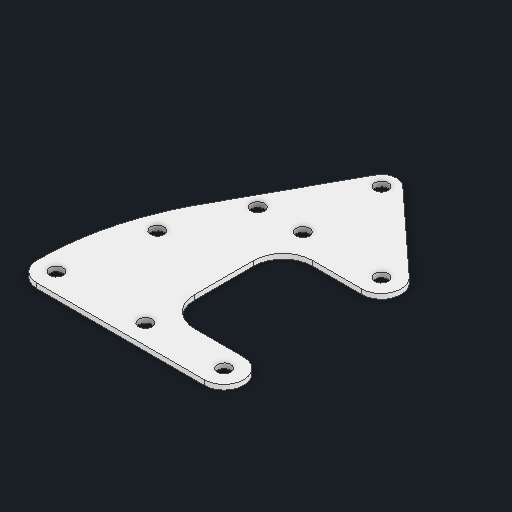
# Autodesk Inventor part: Funnel Gusset Back Improved V2
Saved by Autodesk Inventor 2025.1 (Build 291241000, 241)
## iProperties
Created: 2024-10-23
Part Number: Funnel Gusset Back Improved V2
Material: Acetal Resin, White
Document SubType Name: Modeling
Designer: avere
Density: 1.425 g/cm^3
Appearance: Smooth - White
Author: avere
Autodesk Inventor part; units mm, degrees
ref_plane "YZ Plane" through (0, 0, 0) normal (1, 0, 0) x (0, 1, 0)
ref_plane "XZ Plane" through (0, 0, 0) normal (0, 1, 0) x (-1, 0, 0)
ref_plane "XY Plane" through (0, 0, 0) normal (0, 0, 1) x (1, 0, 0)
sketch "main" plane through (0, 0, 0) normal (0, 0, 1) x (1, 0, 0)
  line L0 (12.0188, -14.2552) -> (33.1027, 24.2387)
  circle A0 centre (21.9619, 13.8124) radius 2.1844
  circle A1 centre (31.5972, 36.5815) radius 2.1844
  circle A2 centre (36.4896, 64.2776) radius 2.1844
  line L1 (36.4904, 70.6276) -> (-17.6528, 70.6344)
  circle A3 centre (7.7473, 64.2844) radius 2.1844
  line L2 (7.7507, 48.4162) -> (7.7558, 29.3619)
  arc A4 (7.7507, 48.4162) -> (-1.7768, 57.9386) centre (-1.7743, 48.4136) ccw
  arc A5 (-1.7692, 19.8344) -> (7.7558, 29.3619) centre (-1.7692, 29.3594) ccw
  line L3 (-17.645, 57.9344) -> (-1.7768, 57.9386)
  arc A6 (-17.6528, 70.6344) -> (-17.645, 57.9344) centre (-17.645, 64.2844) ccw
  arc A7 (-17.6527, 19.8344) -> (-21.9541, 8.8131) centre (-17.6527, 13.4844) ccw
  circle A8 centre (7.7473, 13.4844) radius 2.1844
  line L4 (-1.7692, 19.8344) -> (-17.6527, 19.8344)
  arc A9 (4.4483, -15.4983) -> (12.0188, -14.2552) centre (7.7473, -11.9156) ccw
  line L5 (4.4483, -15.4983) -> (-21.9541, 8.8131)
  circle A10 centre (7.7473, -11.9156) radius 2.1844
  circle A11 centre (-17.645, 64.2844) radius 2.1844
  circle A12 centre (-17.6527, 13.4844) radius 2.1844
  arc A13 (42.8396, 64.2776) -> (36.4904, 70.6276) centre (36.4896, 64.2776) ccw
  arc A14 (33.1027, 24.2387) -> (42.8396, 64.2776) centre (-44.3506, 64.2776) ccw
  point P0 (10.5119, 26.5593)
  dimension "d1" = 9.7405
  dimension "d2" = 4.3688
  dimension "d3" = 4.3688
  dimension "d4" = 4.3688
  dimension "d5" = 4.3688
  dimension "d6" = 4.3688
  dimension "d10" = 50.8
  dimension "d11" = 50.8
  dimension "d13" = 6.35
  measures "d1" diameter of A9
  measures "d2" diameter of A2
  measures "d3" diameter of A3
  measures "d4" diameter of A1
  measures "d5" diameter of A0
  measures "d6" diameter of A8
  measures "d10" distance of A7.centre A11.centre
  measures "d11" distance of A8.centre A3.centre
  measures "d13" radius of A6
sketch "Sketch1" plane through (0, 0, 0) normal (0, 1, 0) x (-1, 0, 0)
  line L0 (29.6638, -78.5396) -> (50.7478, -40.0457)
  circle A0 centre (39.607, -50.472) radius 2.1844
  circle A1 centre (49.2422, -27.7029) radius 2.1844
  circle A2 centre (54.1346, -0.0068) radius 2.1844
  line L1 (54.1354, 6.3432) -> (-0.0077, 6.35)
  circle A3 centre (25.3923, 0) radius 2.1844
  line L2 (25.3957, -15.8682) -> (25.4009, -34.9224)
  arc A4 (25.3957, -15.8682) -> (15.8682, -6.3457) centre (15.8707, -15.8707) ccw
  arc A5 (15.8759, -44.45) -> (25.4009, -34.9224) centre (15.8759, -34.925) ccw
  line L3 (0, -6.35) -> (15.8682, -6.3457)
  arc A6 (-0.0077, 6.35) -> (0, -6.35) centre (0, 0) ccw
  arc A7 (-0.0077, -44.45) -> (-4.309, -55.4713) centre (-0.0077, -50.8) ccw
  circle A8 centre (25.3923, -50.8) radius 2.1844
  line L4 (15.8759, -44.45) -> (-0.0077, -44.45)
  arc A9 (22.0933, -79.7827) -> (29.6638, -78.5396) centre (25.3923, -76.2) ccw
  line L5 (22.0933, -79.7827) -> (-4.309, -55.4713)
  circle A10 centre (25.3923, -76.2) radius 2.1844
  circle A11 centre (0, 0) radius 2.1844
  circle A12 centre (-0.0077, -50.8) radius 2.1844
  arc A13 (60.4846, -0.0068) -> (54.1354, 6.3432) centre (54.1346, -0.0068) ccw
  arc A14 (50.7478, -40.0457) -> (60.4846, -0.0068) centre (-26.7056, -0.0068) ccw
  constraints: 2 other
extrude "Extrusion1" add sketch "Sketch1" along normal blind 1.5875
body "Solid1"
